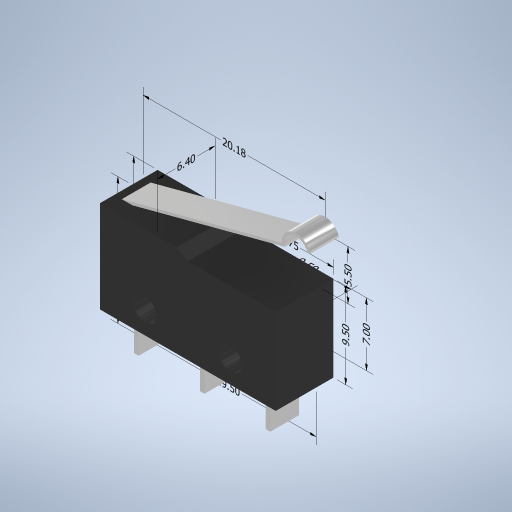
# Autodesk Inventor part: limit_switch
Saved by Autodesk Inventor 2024.1 (Build 281209000, 209)
## iProperties
Created: 2025-01-16
Part Number: limit_switch
Material: アルミニウム 6061
Document SubType Name: Modeling
Designer: hibik
Density: 2.7 g/cm^3
Appearance: アルミニウム - フラット
Author: hibik
Autodesk Inventor part; units mm, degrees
ref_plane "YZ Plane" through (0, 0, 0) normal (1, 0, 0) x (0, 1, 0)
ref_plane "XZ Plane" through (0, 0, 0) normal (0, 1, 0) x (-1, 0, 0)
ref_plane "XY Plane" through (0, 0, 0) normal (0, 0, 1) x (1, 0, 0)
sketch "スケッチ1" plane through (0, 0, 0) normal (0, 0, 1) x (1, 0, 0)
  line L0 (-9.75, 10.2) -> (9.75, 10.2)
  line L1 (9.75, 10.2) -> (9.75, 0)
  line L2 (9.75, 0) -> (-9.75, 0)
  line L3 (-9.75, 0) -> (-9.75, 10.2)
  line L4 (-9.75, 10.2) -> (9.75, 0) construction
  line L5 (9.75, 10.2) -> (-9.75, 0) construction
  line L6 (-13.65, 0) -> (13.65, 0) projected
  point P0 (0, 0)
  point P1 (0, 5.1)
  point P2 (0, 0)
  dimension "d0" = 19.5
  dimension "d1" = 10.2
  constraints: 12 end point, 3 midpoint, 2 parallel, 2 vertical alignment, 1 collinear, 1 horizontal, 1 perpendicular
  measures "d0" distance of L1.end L2.end
  measures "d1" distance of L0.end L1.end
extrude "押し出し1" add sketch "スケッチ1" along normal blind 3.2
sketch "スケッチ2" plane through (0, 0, 3.2) normal (0, 0, 1) x (1, 0, 0)
  line L0 (9.75, 0) -> (9.75, 10.2) projected
  line L1 (9.75, 0) -> (0, 0)
  line L2 (0, 0) -> (0, 9.5)
  line L3 (0, 9.5) -> (9.75, 9.5)
  line L4 (9.75, 9.5) -> (9.75, 0)
  line L5 (-9.75, 0) -> (9.75, 0) projected
  line L6 (0, 9.5) -> (-1.25, 10.2)
  line L7 (9.75, 10.2) -> (-9.75, 10.2) projected
  point P0 (0, 0)
  point P1 (0, 0)
  dimension "d4" = 9.5
  dimension "d5" = 11
  constraints: 10 end point, 2 parallel, 2 point on line, 1 horizontal, 1 midpoint, 1 perpendicular
  measures "d4" distance of L1.end L2.end
  measures "d5" distance from line of L0 L6.end
extrude "押し出し2" cut sketch "スケッチ2" against normal through all contours L3 L6 L7 L0
sketch "スケッチ3" plane through (0, 0, 3.2) normal (0, 0, 1) x (1, 0, 0)
  circle A0 centre (-4.75, 2.5) radius 1.25
  circle A1 centre (4.75, 2.5) radius 1.25
  line L0 (0, -2.04) -> (0, 12.24) projected
  line L1 (-9.75, 0) -> (9.75, 0) projected
  point P0 (0, 0)
  dimension "d8" = 2.5
  dimension "d9" = 9.5
  dimension "d10" = 2.5
  constraints: 2 centre point, 1 equal radius, 1 horizontal alignment, 1 symmetric about line
  measures "d8" diameter of A0
  measures "d9" distance of A0.centre A1.centre
  measures "d10" distance from line of L1 A1.centre
extrude "押し出し3" cut sketch "スケッチ3" against normal through all
sketch "スケッチ5" plane through (0, 0, 0) normal (0, 0, -1) x (-1, 0, 0)
  line L0 (9.75, 0) -> (-9.75, 0) projected
  line L1 (-0.25, 0) -> (0.25, 0)
  line L2 (0.25, 0) -> (0.25, -3.9)
  line L3 (0.25, -3.9) -> (-0.25, -3.9)
  line L4 (-0.25, -3.9) -> (-0.25, 0)
  line L5 (7.05, 0) -> (7.55, 0)
  line L6 (7.55, 0) -> (7.55, -3.9)
  line L7 (7.55, -3.9) -> (7.05, -3.9)
  line L8 (7.05, -3.9) -> (7.05, 0)
  line L9 (-7.55, 0) -> (-7.05, 0)
  line L10 (-7.05, 0) -> (-7.05, -3.9)
  line L11 (-7.05, -3.9) -> (-7.55, -3.9)
  line L12 (-7.55, -3.9) -> (-7.55, 0)
  line L13 (9.75, 0) -> (-9.75, 0) projected
  circle A0 centre (-4.75, 2.5) radius 1.25 projected
  line L14 (-10.4269, 15) -> (-10.3503, 15.2901)
  line L15 (-10.3503, 15.2901) -> (7.8266, 10.4901)
  line L16 (7.8266, 10.4901) -> (7.75, 10.2)
  line L17 (7.75, 10.2) -> (-10.4269, 15)
  line L18 (-11.05, 10.2) -> (7.75, 10.2) construction
  line L19 (1.25, 10.2) -> (9.75, 10.2) projected
  circle A1 centre (4.75, 2.5) radius 1.25 projected
  line L20 (9.75, 10.2) -> (9.75, 0) projected
  arc A2 (-10.4269, 15) -> (-11.05, 10.2) centre (7.75, 10.2) ccw construction
  circle A3 centre (-10.4269, 15) radius 1.3
  circle A4 centre (-10.4269, 15) radius 1.6
  line L21 (-10.4269, 15) -> (-11.9739, 15.4085)
  line L22 (7.8266, 10.4901) -> (8.925, 10.2)
  point P0 (0, 0)
  point P1 (7.3, -3.9)
  point P2 (0, -3.9)
  point P3 (-7.3, -3.9)
  point P4 (0, 0)
  point P5 (-8.8308, 14.8888)
  point P6 (-11.6838, 15.3319)
  point P7 (-9.17, 14.6681)
  dimension "d26" = 3.2
  dimension "d13" = 0.5
  dimension "d14" = 7.3
  dimension "d15" = 7.3
  dimension "d17" = 6.4
  dimension "d21" = 0.3
  dimension "d22" = 15.8
  dimension "d23" = 2
  dimension "d25" = 2.6
  dimension "d27" = 15
  constraints: 38 end point, 9 parallel, 4 equal length, 4 horizontal, 4 midpoint, 4 perpendicular, 3 coincident, 3 collinear, 3 point on line, 2 centre point, 2 point on circle, 1 vertical alignment, 3 other
  measures "d13" distance of L6.end L7.end
  measures "d14" distance of point (7.3, -3.9) point (0, -3.9)
  measures "d15" distance of point (-7.3, -3.9) point (0, -3.9)
  measures "d17" distance from line of L11 A0.centre
  measures "d21" distance between parallel lines of L17 L15
  measures "d22" horizontal distance of L18.start A1.centre
  measures "d23" distance from line of L20 L16.end
  measures "d25" diameter of A3
  measures "d27" distance from line of L14.start L0
extrude "押し出し4" add sketch "スケッチ5" against normal blind 1.6 contours L6 L7 L8 L0 | L2 L3 L4 L0 | L10 L11 L12 L0 | A3 L15 A4 L17 | L21 A4 L15 A3 | A4 L15 L16 L17 | L16 L22 L19
mirror "ミラー1" about plane through (0, 5.1, 0) normal (0, 0, -1)
equation "\"d15\" = d14"
